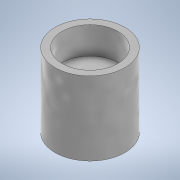
# Autodesk Inventor part: 偏心轮
Saved by Autodesk Inventor 2022 (Build 260153000, 153)
## iProperties
Created: 2022-05-18
Part Number: 偏心轮
Material: 常规
Document SubType Name: Modeling
Designer: zhcne
Density: 1 g/cm^3
Appearance: 默认
Author: zhcne
Autodesk Inventor part; units mm, degrees
ref_plane "YZ Plane" through (0, 0, 0) normal (1, 0, 0) x (0, 1, 0)
ref_plane "XZ Plane" through (0, 0, 0) normal (0, 1, 0) x (-1, 0, 0)
ref_plane "XY Plane" through (0, 0, 0) normal (0, 0, 1) x (1, 0, 0)
sketch "草图1" plane through (0, 0, 0) normal (0, 1, 0) x (-1, 0, 0)
  point P0 (0, 0)
sketch "草图2" plane through (0, 0, 0) normal (0, 1, 0) x (-1, 0, 0)
  circle A0 centre (0, 0) radius 4.5
  arc A1 (-1.4, 1.1619) -> (-1.4, -1.1619) centre (-2.5, 0) ccw
  line L0 (-1.4, 1.1619) -> (-1.4, -1.1619)
  dimension "d0" = 9
  dimension "d1" = 3.2
  dimension "d2" = 2.7
  dimension "d3" = 2.5
  constraints: 2 centre point, 2 end point, 2 point on circle, 1 coincident, 1 horizontal alignment, 1 vertical
  measures "d0" diameter of A0
  measures "d1" diameter of A1
  measures "d3" distance of point (0, 0) A1.centre
extrude "拉伸1" add sketch "草图2" along normal blind 6
sketch "草图3" plane through (0, 6, 0) normal (0, 1, 0) x (1, 0, 0)
  circle A0 centre (0, 0) radius 4.5 projected
  circle A1 centre (0, 0) radius 3.6
  dimension "d6" = 7.2
  constraints: 1 centre point, 1 coincident
  measures "d6" diameter of A1
extrude "拉伸2" add sketch "草图3" along normal blind 3.5
